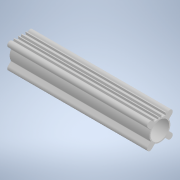
# Autodesk Inventor part: 32-121-200--173-s3
Saved by Autodesk Inventor 2024.3 (Build 283343000, 343)
## iProperties
Category: PARTsolutions
Company: METALWORK
Created: 2025-06-08
Part Number: 32-121-200--173-s3
Material: Generic
Catalog Web Link: www.cadenas.de
Description: ISO 15552 Series 3 barrel-
Vendor: METALWORK
Document SubType Name: Modeling
Designer: psAdmin
Manufacturer: METALWORK
Mass: 159.461 g
Surface Area: 794.183 cm^2
Volume: 159.461 cm^3
Density: 1 g/cm^3
Appearance: PSOLRGB-175-175-175
PSOL_IDENT_0: {$CADENAS_DATA/23d-libs/metalwork/actuators/cyl_ser_iso_15552/series_3_conf/parts/iso_15552_3_barrel
PSOL_IDENT_1: .prj},216 {VTYP=3D},{NB=32-121-200--173-s3},{LINA=32-121-200--173-s3},{NN=ISO 15552 Series 3 barrel}
PSOL_IDENT_2: ,{DATE=21.07.2022 07:22:21},{GEOMDATE=13.04.2018 10:36:00},{VERSION=},{LINEID=10},{WBVAR=TYPE,HUB,VE
PSOL_IDENT_3: R,XV},{WBNUMERIC=HUB,XV}  {NB=32-121-200--173-s3},{LINA=32-121-200--173-s3},{KT=DUMMY},{DI=32},{TYPE=
PSOL_IDENT_4: 121},{TX= '121','Double-acting, cushioned', '122','Through-rod', '124','Double-acting, non-cuschione
PSOL_IDENT_5: d', '125','Opposed', '126','Single-acting', '127','Tandem', '134','Rod lock version', '136','Version
PSOL_IDENT_6: with piston rod lock','137','Piston rod lock + guide unit' },{HUB=200},{VER=},{VERX='','N/A'},{L0=9
PSOL_IDENT_7: 4.000},{HL1=26.000},{XV=173.0},{XDEF=173.000},{XMIN=63.000},{XMAX=283.000},{WH=26.000},{SY=19.650},{
PSOL_IDENT_8: SZ=6.500},{X=6.50},{Y=17.60}
NB: 32-121-200--173-s3
NN: ISO 15552 Series 3 barrel
NBSYN: $DI.-$TYPE.-$HUB.-$VER.-$XV.-s3
LINA: 32-121-200--173-s3
CATALOG: Metalwork
DI: 32
TYPE: Double-acting, cushioned
HUB: 200
VER: N/A
HL1: 26
XV: 173
XMIN: 63
WH: 26
SY: 19.65
SZ: 6.5
X: 6.5
Y: 17.6
SUPPLIER: METALWORK
ARTICLENO: 32-121-200--173-s3
BOMINFO: 32-121-200--173-s3
CREATOR: CADENAS GmbH
Title: 32-121-200--173-s3
Author: Cadenas PARTsolutions
Autodesk Inventor part; units mm, degrees
sketch "Sketch_1" plane through (0, 0, 0) normal (1, 0, 0) x (0, 1, 0)
  arc A0 (-14.0912, 20.8088) -> (-20.8088, 14.0912) centre (-17.45, 17.45) ccw
  line L0 (-20.8088, 14.0912) -> (-16.1638, 9.4463)
  arc A1 (-15.9829, 8.2792) -> (-16.1638, 9.4463) centre (-16.8709, 8.7392) ccw
  arc A2 (-15.9829, 8.2792) -> (-15.983, -8.2792) centre (0, 0) ccw
  arc A3 (-16.1638, -9.4463) -> (-15.983, -8.2792) centre (-16.8709, -8.7392) ccw
  line L1 (-16.1638, -9.4463) -> (-20.8088, -14.0912)
  arc A4 (-20.8088, -14.0912) -> (-14.0912, -20.8088) centre (-17.45, -17.45) ccw
  line L2 (-14.0912, -20.8088) -> (-9.4463, -16.1638)
  arc A5 (-8.2792, -15.9829) -> (-9.4463, -16.1638) centre (-8.7392, -16.8709) ccw
  arc A6 (-8.2792, -15.9829) -> (8.2792, -15.983) centre (0, 0) ccw
  arc A7 (9.4463, -16.1638) -> (8.2792, -15.983) centre (8.7392, -16.8709) ccw
  line L3 (9.4463, -16.1638) -> (14.0912, -20.8088)
  arc A8 (14.0912, -20.8088) -> (20.8088, -14.0912) centre (17.45, -17.45) ccw
  line L4 (20.8088, -14.0912) -> (18.7215, -12.004)
  arc A9 (18.8549, -11.581) -> (18.7215, -12.004) centre (18.8983, -11.8272) ccw
  line L5 (18.8549, -11.581) -> (21.6129, -11.0947)
  arc A10 (21.6129, -11.0947) -> (22.15, -10.4546) centre (21.5, -10.4546) ccw
  line L6 (22.15, -10.4546) -> (22.15, -9.625)
  arc A11 (22.15, -9.625) -> (21.75, -9.225) centre (21.75, -9.625) ccw
  line L7 (21.75, -9.225) -> (20.9499, -9.225)
  line L8 (20.9499, -9.225) -> (20.9499, -9.9)
  line L9 (20.9499, -9.9) -> (17.9999, -9.9)
  arc A12 (17.5999, -9.5) -> (17.9999, -9.9) centre (17.9999, -9.5) ccw
  line L10 (17.5999, -9.5) -> (17.5999, -3.5)
  arc A13 (17.9999, -3.1) -> (17.5999, -3.5) centre (17.9999, -3.5) ccw
  line L11 (17.9999, -3.1) -> (20.9499, -3.1)
  line L12 (20.9499, -3.1) -> (20.9499, -3.775)
  line L13 (20.9499, -3.775) -> (21.75, -3.775)
  arc A14 (21.75, -3.775) -> (22.15, -3.375) centre (21.75, -3.375) ccw
  line L14 (22.15, -3.375) -> (22.15, -2.5454)
  arc A15 (22.15, -2.5454) -> (21.6129, -1.9053) centre (21.5, -2.5454) ccw
  line L15 (21.6129, -1.9053) -> (18.3939, -1.3377)
  arc A16 (17.9812, -0.8224) -> (18.3939, -1.3377) centre (18.4807, -0.8453) ccw
  arc A17 (17.9812, -0.8224) -> (17.9812, 0.8224) centre (0, 0) ccw
  arc A18 (18.3939, 1.3377) -> (17.9812, 0.8224) centre (18.4807, 0.8453) ccw
  line L16 (18.3939, 1.3377) -> (21.6129, 1.9053)
  arc A19 (21.6129, 1.9053) -> (22.15, 2.5454) centre (21.5, 2.5454) ccw
  line L17 (22.15, 2.5454) -> (22.15, 3.375)
  arc A20 (22.15, 3.375) -> (21.75, 3.775) centre (21.75, 3.375) ccw
  line L18 (21.75, 3.775) -> (20.9499, 3.775)
  line L19 (20.9499, 3.775) -> (20.9499, 3.1)
  line L20 (20.9499, 3.1) -> (17.9999, 3.1)
  arc A21 (17.5999, 3.5) -> (17.9999, 3.1) centre (17.9999, 3.5) ccw
  line L21 (17.5999, 3.5) -> (17.5999, 9.5)
  arc A22 (17.9999, 9.9) -> (17.5999, 9.5) centre (17.9999, 9.5) ccw
  line L22 (17.9999, 9.9) -> (20.9499, 9.9)
  line L23 (20.9499, 9.9) -> (20.9499, 9.225)
  line L24 (20.9499, 9.225) -> (21.75, 9.225)
  arc A23 (21.75, 9.225) -> (22.15, 9.625) centre (21.75, 9.625) ccw
  line L25 (22.15, 9.625) -> (22.15, 10.4546)
  arc A24 (22.15, 10.4546) -> (21.6129, 11.0947) centre (21.5, 10.4546) ccw
  line L26 (21.6129, 11.0947) -> (18.8549, 11.581)
  arc A25 (18.7215, 12.004) -> (18.8549, 11.581) centre (18.8983, 11.8272) ccw
  line L27 (18.7215, 12.004) -> (20.8088, 14.0912)
  arc A26 (20.8088, 14.0912) -> (14.0912, 20.8088) centre (17.45, 17.45) ccw
  line L28 (14.0912, 20.8088) -> (9.4463, 16.1638)
  arc A27 (8.2792, 15.983) -> (9.4463, 16.1638) centre (8.7392, 16.8709) ccw
  arc A28 (8.2792, 15.983) -> (-8.2792, 15.983) centre (0, 0) ccw
  arc A29 (-9.4463, 16.1638) -> (-8.2792, 15.983) centre (-8.7392, 16.8709) ccw
  line L29 (-9.4463, 16.1638) -> (-14.0912, 20.8088)
  circle A30 centre (0, 0) radius 16
  constraints: 60 end point, 60 point on circle, 31 centre point
extrude "Extrusion1" add sketch "Sketch_1" along normal blind 242
ref_plane "br_l_XY" through (0, 0, 0) normal (1, 0, 0) x (0, 0, -1)
ref_plane "br_l_YZ" through (0, 0, 0) normal (0, 0, -1) x (0, 1, 0)
ref_plane "br_l_ZX" through (0, 0, 0) normal (0, 1, 0) x (1, 0, 0)
ref_plane "br_r_XY" through (242, 0, 0) normal (-1, 0, 0) x (0, 0, -1)
ref_plane "br_r_YZ" through (242, 0, 0) normal (0, 0, -1) x (0, -1, 0)
ref_plane "br_r_ZX" through (242, 0, 0) normal (0, -1, 0) x (-1, 0, 0)
ref_plane "mod_en_XY" through (121, 0, 0) normal (1, 0, 0) x (0, 0, -1)
ref_plane "mod_en_YZ" through (121, 0, 0) normal (0, 0, -1) x (0, 1, 0)
ref_plane "mod_en_ZX" through (121, 0, 0) normal (0, 1, 0) x (1, 0, 0)
ref_plane "sens_sqr_l_XY" through (0, 17.6, -6.5) normal (-1, 0, 0) x (0, 0, -1)
ref_plane "sens_sqr_l_YZ" through (0, 17.6, -6.5) normal (0, 0, -1) x (0, -1, 0)
ref_plane "sens_sqr_l_ZX" through (0, 17.6, -6.5) normal (0, -1, 0) x (-1, 0, 0)
ref_plane "sens_sqr_r_XY" through (242, 17.6, 6.5) normal (1, 0, 0) x (0, 0, -1)
ref_plane "sens_sqr_r_YZ" through (242, 17.6, 6.5) normal (0, 0, -1) x (0, 1, 0)
ref_plane "sens_sqr_r_ZX" through (242, 17.6, 6.5) normal (0, 1, 0) x (1, 0, 0)
ref_plane "sensor_l_XY" through (2.7, 19.65, -6.5) normal (0, -1, 0) x (1, 0, 0)
ref_plane "sensor_l_YZ" through (2.7, 19.65, -6.5) normal (1, 0, 0) x (0, 0, 1)
ref_plane "sensor_l_ZX" through (2.7, 19.65, -6.5) normal (0, 0, 1) x (0, -1, 0)
ref_plane "sensor_r_XY" through (239.3, 19.65, 6.5) normal (0, -1, 0) x (1, 0, 0)
ref_plane "sensor_r_YZ" through (239.3, 19.65, 6.5) normal (1, 0, 0) x (0, 0, 1)
ref_plane "sensor_r_ZX" through (239.3, 19.65, 6.5) normal (0, 0, 1) x (0, -1, 0)
body "Solid1"
